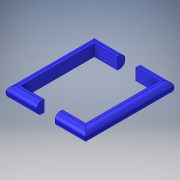
# Autodesk Inventor part: Bumbers.ver1-1111-2019
Saved by Autodesk Inventor 2018 (Build 220112000, 112)
## iProperties
Created: 2020-01-06
Part Number: Bumbers.ver1-1111-2019
Material: Nylon 6/6
Document SubType Name: Modeling
Designer: JMHal
Density: 1.13 g/cm^3
Appearance: Nylon 6
Author: JMHal
Autodesk Inventor part; units mm, degrees
ref_plane "YZ Plane" through (0, 0, 0) normal (1, 0, 0) x (0, 1, 0)
ref_plane "XZ Plane" through (0, 0, 0) normal (0, 1, 0) x (-1, 0, 0)
sketch "Sketch1" plane through (0, 0, 0) normal (0, 1, 0) x (-1, 0, 0)
  line L0 (0, 0) -> (717.55, 0)
  line L1 (717.55, 0) -> (717.55, -812.8)
  line L2 (717.55, -812.8) -> (0, -812.8)
  line L3 (0, -812.8) -> (0, 0)
  line L4 (800.1, -895.35) -> (800.1, 82.55)
  line L5 (800.1, 82.55) -> (-82.55, 82.55)
  line L6 (-82.55, 82.55) -> (-82.55, -895.35)
  line L7 (-82.55, -895.35) -> (800.1, -895.35)
  dimension "d0" = 812.8
  dimension "d1" = 717.55
  dimension "d2" = 82.55
  constraints: 16 end point, 4 parallel, 2 perpendicular, 1 horizontal, 3 other
  measures "d0" distance of L0.end L1.end
  measures "d1" distance of L1.end L2.end
  measures "d2" distance between parallel lines of L1 L4
extrude "Extrusion1" add sketch "Sketch1" along normal blind 127
fillet "Fillet1" radius 57.15 8 edges at (82.55, 127, -406.4) (82.55, 0, -406.4) (-358.775, 0, 82.55) (-358.775, 127, 82.55) (-358.775, 127, -895.35) (-358.775, 0, -895.35) (-800.1, 127, -406.4) (-800.1, 0, -406.4)
sketch "Sketch2" plane through (0, 0, 0) normal (0, 0, -1) x (-1, 0, 0)
  line L0 (717.55, 0) -> (0, 0) projected
  line L1 (717.55, 0) -> (717.55, 127) projected
  line L2 (0, 127) -> (717.55, 127) projected
  line L3 (0, 0) -> (0, 127) projected
  line L4 (460.375, 127) -> (460.375, 0)
  line L5 (717.55, 0) -> (0, 0) projected
  line L6 (0, 127) -> (717.55, 127) projected
  line L7 (257.175, 127) -> (257.175, 0)
  line L8 (358.775, 0) -> (358.775, 127)
  dimension "d6" = 203.2
  constraints: 6 end point, 4 point on line, 2 midpoint, 1 perpendicular, 1 vertical, 1 other
  measures "d6" distance between parallel lines of L4 L7
extrude "Extrusion2" cut sketch "Sketch2" against normal blind 127 contours L0 L8 L2 L4 | L0 L7 L2 L8
ref_plane "Work Plane1" through (-800.1, 57.15, -406.4) normal (0, 0, 1) x (1, 0, 0)
mirror "Mirror1" about plane through (-800.1, 57.15, -406.4) normal (0, 0, 1) of "Extrusion2"
body "Solid1"
